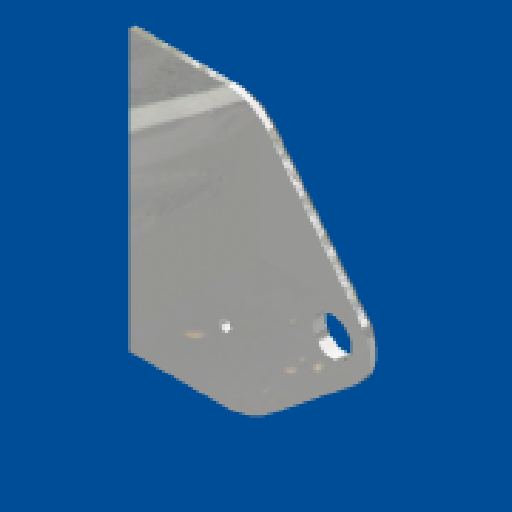
# Autodesk Inventor part: baseOuter
Saved by Autodesk Inventor 2023 (Build 270158030, 158C)
## iProperties
Created: 2023-03-03
Part Number: baseOuter
Material: Aluminum 6061
Document SubType Name: Modeling
Designer: kumpu
Mass: 219.441 g
Surface Area: 289.319 cm^2
Volume: 81.2743 cm^3
Density: 2.7 g/cm^3
Appearance: Aluminum - Dark
Author: kumpu
Autodesk Inventor part; units mm, degrees
ref_plane "YZ Plane" through (0, 0, 0) normal (1, 0, 0) x (0, 1, 0)
ref_plane "XZ Plane" through (0, 0, 0) normal (0, 1, 0) x (-1, 0, 0)
ref_plane "XY Plane" through (0, 0, 0) normal (0, 0, 1) x (1, 0, 0)
sketch "Sketch1" plane through (0, 0, 0) normal (0, 0, 1) x (1, 0, 0)
  line L0 (0, 0) -> (49.2125, 0)
  arc A0 (69.2791, -9.8278) -> (49.2125, 0) centre (49.2125, -25.4) ccw
  line L1 (69.2791, -9.8278) -> (116.6499, -70.8709)
  arc A1 (113.4684, -97.4512) -> (116.6499, -70.8709) centre (101.6, -82.55) ccw
  line L2 (113.4684, -97.4512) -> (70.102, -131.9913)
  arc A2 (48.0501, -139.7) -> (70.102, -131.9913) centre (48.0501, -104.3043) ccw
  line L3 (48.0501, -139.7) -> (0, -139.7)
  line L4 (0, -139.7) -> (0, 0)
  line L5 (0, -139.7) -> (12.7, -139.7) construction
  circle A3 centre (101.6, -82.55) radius 16 construction
  circle A4 centre (48.0501, -104.3043) radius 7.025 construction
  arc A5 (33.057, -35.4) -> (32.0953, -33.6463) centre (49.2125, -25.4) ccw construction
  circle A6 centre (38.1, -63.5) radius 17.907 construction
  circle A7 centre (71.7198, -40.8503) radius 7.025 construction
  circle A8 centre (38.1, -63.5) radius 19.05
  circle A9 centre (48.0501, -104.3043) radius 3
  circle A10 centre (101.6, -82.55) radius 9.525
  dimension "d0" = 19.05
  dimension "d1" = 38.1
  dimension "d4" = 6
  dimension "d5" = 19.05
  constraints: 10 end point, 6 centre point, 6 coincident, 6 point on circle, 6 tangent, 1 collinear, 1 horizontal, 1 parallel, 1 perpendicular
  measures "d0" radius of A1
  measures "d1" diameter of A8
  measures "d4" diameter of A9
  measures "d5" diameter of A10
extrude "Extrusion1" add sketch "Sketch1" along normal blind 6.35 contours L0 A0 L1 A1 L2 A2 L3 L4 | A8
chamfer "Chamfer1" distance 3.175 angle 45 7 edges at (92.9645, -40.3494, 0) (60.3845, -2.5889, 0) (24.6062, 0, 0) (120.515, -84.8141, 0) (91.7852, -114.7212, 0) (59.7304, -137.7173, 0) (24.0251, -139.7, 0)
body "Solid1"
